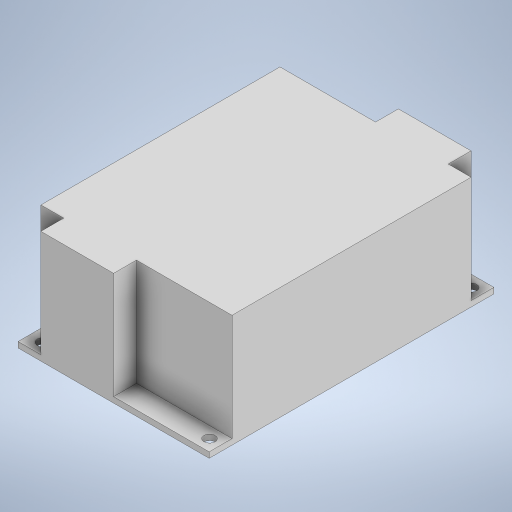
# Autodesk Inventor part: 24V
Saved by Autodesk Inventor 2023 (Build 270158000, 158)
## iProperties
Created: 2022-04-18
Part Number: 24V
Material: Generic
Document SubType Name: Modeling
Designer: benni
Density: 1 g/cm^3
Appearance: Default
Author: benni
Autodesk Inventor part; units mm, degrees
ref_plane "YZ Plane" through (0, 0, 0) normal (1, 0, 0) x (0, 1, 0)
ref_plane "XZ Plane" through (0, 0, 0) normal (0, 1, 0) x (-1, 0, 0)
ref_plane "XY Plane" through (0, 0, 0) normal (0, 0, 1) x (1, 0, 0)
sketch "Sketch1" plane through (0, 0, 0) normal (0, 1, 0) x (-1, 0, 0)
  line L0 (0, 0) -> (51, 0)
  line L1 (51, 0) -> (51, -76)
  line L2 (51, -76) -> (0, -76)
  line L3 (0, -76) -> (0, 0)
  line L4 (25.2419, 25.0701) -> (25.2419, -108.9673)
  line L5 (67.6146, -38) -> (-16.7983, -38)
  circle A0 centre (47.4919, -3.1) radius 1.5
  line L6 (25.2419, -101.0701) -> (25.2419, 32.9673)
  circle A1 centre (47.4919, -72.9) radius 1.5
  circle A2 centre (2.9919, -3.1) radius 1.5
  circle A3 centre (2.9919, -72.9) radius 1.5
  line L7 (0, -6.6687) -> (0, -69.6719)
  line L8 (51, -69.6719) -> (51, -6.6687)
  line L9 (43.5757, 0) -> (25.2419, 0)
  line L10 (25.2419, 0) -> (25.2419, -6.6687)
  line L11 (25.2419, -69.6719) -> (25.2419, -76)
  line L12 (25.2419, -76) -> (6.2363, -76)
  point P0 (25.2419, 0)
  point P1 (25.2419, -76)
  dimension "d0" = 51
  dimension "d1" = 76
  dimension "d2" = 69.8
  dimension "d3" = 44.5
  dimension "d4" = 3
  dimension "d11" = 3.1
  constraints: 26 end point, 8 symmetric about line, 6 point on line, 4 centre point, 3 horizontal, 3 parallel, 2 perpendicular, 1 coincident, 1 vertical, 3 other
  measures "d0" distance of L1.end L2.end
  measures "d1" distance of L0.end L1.end
  measures "d2" diameter of point (47.492, -3.1) L5
  measures "d3" diameter of point (47.492, -3.1) L4
  measures "d4" diameter of A0
  measures "d11" distance from line of L0 A2.centre
extrude "Extrusion2" add sketch "Sketch1" along normal blind 1.5
sketch "Sketch2" plane through (0, 1.5, 0) normal (0, 1, 0) x (1, 0, 0)
  line L0 (0, 76) -> (-51, 76) projected
  line L1 (-25.5, 76) -> (-6.1, 76)
  line L2 (-6.1, 76) -> (-6.1, 6.1)
  line L3 (-6.1, 6.1) -> (-25.5, 6.1)
  line L4 (-25.5, 6.1) -> (-25.5, 76)
  circle A0 centre (-2.9919, 3.1) radius 1.5 projected
  line L5 (0, 0) -> (0, 76) projected
  line L6 (-51, 76) -> (-51, 0) projected
  line L7 (-51, 69.9) -> (-44.9, 69.9)
  line L8 (-44.9, 69.9) -> (-44.9, 6.1)
  line L9 (-44.9, 6.1) -> (-51, 6.1)
  line L10 (-51, 6.1) -> (-51, 69.9)
  line L11 (-6.1, 69.9) -> (0, 69.9)
  line L12 (0, 69.9) -> (0, 6.1)
  line L13 (0, 6.1) -> (-6.1, 6.1)
  line L14 (-6.1, 6.1) -> (-6.1, 69.9)
  line L15 (-51, 0) -> (0, 0) projected
  line L16 (-25.5, 0) -> (-44.9, 0)
  line L17 (-44.9, 0) -> (-44.9, 69.9)
  line L18 (-44.9, 69.9) -> (-25.5, 69.9)
  line L19 (-25.5, 69.9) -> (-25.5, 0)
  point P0 (-47.95, 6.1)
  point P1 (-47.95, 69.9)
  point P2 (-44.9, 6.1)
  point P3 (-6.1, 6.1)
  point P4 (0, 69.9)
  point P5 (-6.1, 76)
  dimension "d12" = 6.1
  dimension "d14" = 6.1
  dimension "d15" = 6.1
  dimension "d16" = 6.1
  dimension "d17" = 6.1
  dimension "d18" = 6.1
  constraints: 32 end point, 8 parallel, 4 horizontal, 4 midpoint, 4 perpendicular, 3 point on line
  measures "d12" distance between parallel lines of L5 L2
  measures "d14" distance between parallel lines of L6 L17
  measures "d15" distance from line of L15 point (-47.95, 6.1)
  measures "d16" distance from line of L0 point (-47.95, 69.9)
  measures "d17" distance between parallel lines of L0 L18
  measures "d18" distance between parallel lines of L0 L11
extrude "Extrusion3" add sketch "Sketch2" along normal blind 28.5 contours L2 L3 L4 L0 | L5 L13 L2 L11 | L4 L19 L15 L17 L8 L18 | L7 L8 L9 L6
body "Solid2"
